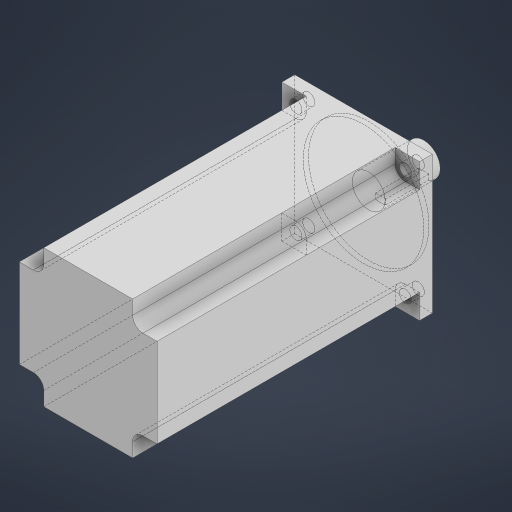
# Autodesk Inventor part: 80AST-A1C02430
Saved by Autodesk Inventor 2023 (Build 270158000, 158)
## iProperties
Created: 2025-09-03
Part Number: 80AST-A1C02430
Material: 일반
Document SubType Name: Modeling
Designer: k
Density: 1 g/cm^3
Appearance: 기본값
Author: k
Autodesk Inventor part; units mm, degrees
ref_plane "YZ Plane" through (0, 0, 0) normal (1, 0, 0) x (0, 1, 0)
ref_plane "XZ Plane" through (0, 0, 0) normal (0, 1, 0) x (-1, 0, 0)
ref_plane "XY Plane" through (0, 0, 0) normal (0, 0, 1) x (1, 0, 0)
sketch "스케치1" plane through (0, 0, 0) normal (0, 0, 1) x (1, 0, 0)
  line L0 (-17.2003, 14.1332) -> (62.7997, 14.1332)
  line L1 (62.7997, 14.1332) -> (62.7997, -65.8668)
  line L2 (62.7997, -65.8668) -> (-17.2003, -65.8668)
  line L3 (-17.2003, -65.8668) -> (-17.2003, 14.1332)
  circle A0 centre (-9.0201, 5.953) radius 3.5
  circle A1 centre (-9.0201, -57.6866) radius 3.5
  circle A2 centre (54.6195, -57.6866) radius 3.5
  circle A3 centre (54.6195, 5.953) radius 3.5
  point P0 (0, 0)
  dimension "d0" = 80
  dimension "d1" = 80
  dimension "d3" = 7
  dimension "d4" = 7
  constraints: 8 end point, 4 centre point, 2 parallel, 1 horizontal, 1 perpendicular
  measures "d0" distance of L1.end L2.end
  measures "d1" distance of L0.end L1.end
  measures "d3" diameter of A0
  measures "d4" diameter of A1
extrude "돌출1" add sketch "스케치1" along normal blind 7.5
sketch "스케치2" plane through (0, 0, 7.5) normal (0, 0, 1) x (1, 0, 0)
  circle A0 centre (-9.0201, 5.953) radius 3.5 projected
  circle A1 centre (-9.0201, 5.953) radius 6
  circle A2 centre (54.6195, -57.6866) radius 3.5 projected
  circle A3 centre (54.6195, -57.6866) radius 6
  circle A4 centre (-9.0201, -57.6866) radius 6
  circle A5 centre (54.6195, 5.953) radius 6
  line L0 (62.7997, 14.1332) -> (-17.2003, 14.1332) projected
  line L1 (-17.2003, 14.1332) -> (-17.2003, -65.8668) projected
  line L2 (-3.0201, 5.953) -> (-3.0201, 15.0573)
  line L3 (-9.0201, -0.047) -> (-23.8178, -0.047)
  line L4 (-9.0201, -51.6866) -> (-23.8178, -51.6866)
  line L5 (-3.0201, -57.6866) -> (-3.0201, -70.3063)
  line L6 (54.6195, -51.6866) -> (67.4303, -51.6866)
  line L7 (48.6195, -57.6866) -> (48.6195, -69.0071)
  line L8 (48.6195, 5.953) -> (48.6195, 16.5093)
  line L9 (54.6195, -0.047) -> (71.0221, -0.047)
  line L10 (-17.2003, -0.047) -> (-17.2003, -51.6866)
  line L11 (-17.2003, -65.8668) -> (62.7997, -65.8668) projected
  line L12 (-3.0201, -65.8668) -> (48.6195, -65.8668)
  line L13 (62.7997, -65.8668) -> (62.7997, 14.1332) projected
  line L14 (62.7997, -51.6866) -> (62.7997, -0.047)
  line L15 (48.6195, 14.1332) -> (-3.0201, 14.1332)
  point P0 (0, 0)
  dimension "d7" = 12
  dimension "d8" = 12
  dimension "d9" = 12
  dimension "d10" = 12
  constraints: 24 end point, 16 point on line, 8 point on circle, 4 centre point, 4 horizontal, 3 perpendicular, 3 tangent, 2 coincident, 1 vertical
  measures "d7" diameter of A1
  measures "d8" diameter of A3
  measures "d9" diameter of A4
  measures "d10" diameter of A5
extrude "돌출2" add sketch "스케치2" along normal blind 152.5 contours L2 L0 L8 A5 L9 L13 L6 A3 L7 L11 L5 A4 L4 L1 L3 A1
sketch "스케치3" plane through (0, 0, 0) normal (0, 0, -1) x (-1, 0, 0)
  circle A0 centre (-22.7997, -25.8668) radius 35
  line L0 (17.2003, 14.1332) -> (17.2003, -65.8668) projected
  line L1 (17.2003, -65.8668) -> (-62.7997, -65.8668) projected
  point P0 (0, 0)
  dimension "d13" = 70
  dimension "d14" = 40
  dimension "d15" = 40
  constraints: 1 centre point
  measures "d13" diameter of A0
  measures "d14" distance from line of L0 A0.centre
  measures "d15" distance from line of L1 A0.centre
extrude "돌출3" add sketch "스케치3" along normal blind 3
sketch "스케치4" plane through (22.7997, -25.8668, -3) normal (0, 0, -1) x (-1, 0, 0)
  point P0 (22.7997, 25.8668)
sketch "스케치5" plane through (22.7997, -25.8668, -3) normal (0, 0, -1) x (-1, 0, 0)
  circle A0 centre (0, 0) radius 35 projected
  circle A1 centre (0, 0) radius 9.5
  point P0 (22.7997, 25.8668)
  dimension "d18" = 19
  constraints: 1 centre point, 1 coincident
  measures "d18" diameter of A1
extrude "돌출4" add sketch "스케치5" along normal blind 32 contours A1
sketch "스케치6" plane through (22.7997, -25.8668, -35) normal (0, 0, -1) x (-1, 0, 0)
  line L0 (3, -20.6113) -> (3, -6)
  line L1 (3, -6) -> (-3, -6)
  line L2 (-3, -6) -> (-3, -20.6113)
  circle A0 centre (0, 0) radius 9.5 projected
  point P0 (22.7997, 25.8668)
  point P1 (-3, -13.3057)
  point P2 (-3, -9.0139)
  point P3 (3, -9.0139)
  dimension "d21" = 15.5
  dimension "d22" = 6
  dimension "d23" = 3
  constraints: 6 end point, 2 perpendicular, 1 midpoint, 1 vertical
  measures "d22" distance from line of point (-3, -13.306) L0
  measures "d23" distance from line of A0.centre L0
extrude "돌출5" cut sketch "스케치6" against normal blind 25 contours A0 L2 L1 L0 picked at (0.3385, -7.1485)
